Autodesk Fusion 360 part; units mm, degrees
note: some values were not read from the file. Chosen so that the rebuilt part matches the saved one: which face or edge a step refers to. Set by a fixed rule: which sketch regions a step uses.
(part 2 of 2)
sketch "Skizze1 (3)" plane through (0, 0, 8) normal (0, 0, 1) x (1, 0, 0) in component "Component''"
  arc A0 (-8, 3) -> (-3, -2) centre (-3, 3) ccw
  line L0 (-3, -2) -> (42, -2)
  arc A1 (42, -2) -> (47, 3) centre (42, 3) ccw
  line L1 (47, 3) -> (47, 46.6)
  arc A2 (47, 46.6) -> (42, 51.6) centre (42, 46.6) ccw
  line L2 (42, 51.6) -> (-3, 51.6)
  arc A3 (-3, 51.6) -> (-8, 46.6) centre (-3, 46.6) ccw
  line L3 (-8, 46.6) -> (-8, 3)
  circle A4 centre (42.5, 2.5) radius 1.5
  line L4 (36.6, 34.1) -> (36.1, 34.1)
  line L5 (36.1, 34.1) -> (36.1, 41.1)
  line L6 (36.1, 41.1) -> (28.8, 41.1)
  line L7 (28.8, 41.1) -> (28.8, 34.1)
  line L8 (28.8, 34.1) -> (28.3, 34.1)
  line L9 (28.3, 34.1) -> (28.3, 41.6)
  line L10 (28.3, 41.6) -> (36.6, 41.6)
  line L11 (36.6, 41.6) -> (36.6, 34.1)
  line L12 (27.1, 34.1) -> (26.6, 34.1)
  line L13 (26.6, 34.1) -> (26.6, 41.1)
  line L14 (26.6, 41.1) -> (19.3, 41.1)
  line L15 (19.3, 41.1) -> (19.3, 34.1)
  line L16 (19.3, 34.1) -> (18.8, 34.1)
  line L17 (18.8, 34.1) -> (18.8, 41.6)
  line L18 (18.8, 41.6) -> (27.1, 41.6)
  line L19 (27.1, 41.6) -> (27.1, 34.1)
  line L20 (17.6, 34.1) -> (17.1, 34.1)
  line L21 (17.1, 34.1) -> (17.1, 41.1)
  line L22 (17.1, 41.1) -> (9.8, 41.1)
  line L23 (9.8, 41.1) -> (9.8, 34.1)
  line L24 (9.8, 34.1) -> (9.3, 34.1)
  line L25 (9.3, 34.1) -> (9.3, 41.6)
  line L26 (9.3, 41.6) -> (17.6, 41.6)
  line L27 (17.6, 41.6) -> (17.6, 34.1)
  circle A5 centre (-3.5, 2.5) radius 1.5
  circle A6 centre (42.5, 47.1) radius 1.5
  circle A7 centre (-3.5, 47.1) radius 1.5
  line L28 (17.6, 7.6) -> (17.1, 7.6)
  line L29 (17.1, 7.6) -> (17.1, 14.6)
  line L30 (17.1, 14.6) -> (9.8, 14.6)
  line L31 (9.8, 14.6) -> (9.8, 7.6)
  line L32 (9.8, 7.6) -> (9.3, 7.6)
  line L33 (9.3, 7.6) -> (9.3, 15.1)
  line L34 (9.3, 15.1) -> (17.6, 15.1)
  line L35 (17.6, 15.1) -> (17.6, 7.6)
  line L36 (27.1, 7.6) -> (26.6, 7.6)
  line L37 (26.6, 7.6) -> (26.6, 14.6)
  line L38 (26.6, 14.6) -> (19.3, 14.6)
  line L39 (19.3, 14.6) -> (19.3, 7.6)
  line L40 (19.3, 7.6) -> (18.8, 7.6)
  line L41 (18.8, 7.6) -> (18.8, 15.1)
  line L42 (18.8, 15.1) -> (27.1, 15.1)
  line L43 (27.1, 15.1) -> (27.1, 7.6)
  line L44 (17.6, 25.2667) -> (17.1, 25.2667)
  line L45 (17.1, 25.2667) -> (17.1, 32.2667)
  line L46 (17.1, 32.2667) -> (9.8, 32.2667)
  line L47 (9.8, 32.2667) -> (9.8, 25.2667)
  line L48 (9.8, 25.2667) -> (9.3, 25.2667)
  line L49 (9.3, 25.2667) -> (9.3, 32.7667)
  line L50 (9.3, 32.7667) -> (17.6, 32.7667)
  line L51 (17.6, 32.7667) -> (17.6, 25.2667)
  line L52 (36.6, 7.6) -> (36.1, 7.6)
  line L53 (36.1, 7.6) -> (36.1, 14.6)
  line L54 (36.1, 14.6) -> (28.8, 14.6)
  line L55 (28.8, 14.6) -> (28.8, 7.6)
  line L56 (28.8, 7.6) -> (28.3, 7.6)
  line L57 (28.3, 7.6) -> (28.3, 15.1)
  line L58 (28.3, 15.1) -> (36.6, 15.1)
  line L59 (36.6, 15.1) -> (36.6, 7.6)
  line L60 (-0.2, 41.6) -> (8.1, 41.6)
  line L61 (8.1, 41.6) -> (8.1, 34.1)
  line L62 (8.1, 34.1) -> (7.6, 34.1)
  line L63 (7.6, 34.1) -> (7.6, 41.1)
  line L64 (7.6, 41.1) -> (0.3, 41.1)
  line L65 (0.3, 41.1) -> (0.3, 34.1)
  line L66 (0.3, 34.1) -> (-0.2, 34.1)
  line L67 (-0.2, 34.1) -> (-0.2, 41.6)
  line L68 (8.1, 25.2667) -> (7.6, 25.2667)
  line L69 (7.6, 25.2667) -> (7.6, 32.2667)
  line L70 (7.6, 32.2667) -> (0.3, 32.2667)
  line L71 (0.3, 32.2667) -> (0.3, 25.2667)
  line L72 (0.3, 25.2667) -> (-0.2, 25.2667)
  line L73 (-0.2, 25.2667) -> (-0.2, 32.7667)
  line L74 (-0.2, 32.7667) -> (8.1, 32.7667)
  line L75 (8.1, 32.7667) -> (8.1, 25.2667)
  line L76 (8.1, 16.4333) -> (7.6, 16.4333)
  line L77 (7.6, 16.4333) -> (7.6, 23.4333)
  line L78 (7.6, 23.4333) -> (0.3, 23.4333)
  line L79 (0.3, 23.4333) -> (0.3, 16.4333)
  line L80 (0.3, 16.4333) -> (-0.2, 16.4333)
  line L81 (-0.2, 16.4333) -> (-0.2, 23.9333)
  line L82 (-0.2, 23.9333) -> (8.1, 23.9333)
  line L83 (8.1, 23.9333) -> (8.1, 16.4333)
  line L84 (8.1, 7.6) -> (7.6, 7.6)
  line L85 (7.6, 7.6) -> (7.6, 14.6)
  line L86 (7.6, 14.6) -> (0.3, 14.6)
  line L87 (0.3, 14.6) -> (0.3, 7.6)
  line L88 (0.3, 7.6) -> (-0.2, 7.6)
  line L89 (-0.2, 7.6) -> (-0.2, 15.1)
  line L90 (-0.2, 15.1) -> (8.1, 15.1)
  line L91 (8.1, 15.1) -> (8.1, 7.6)
  line L92 (36.6, 16.4333) -> (36.1, 16.4333)
  line L93 (36.1, 16.4333) -> (36.1, 23.4333)
  line L94 (36.1, 23.4333) -> (28.8, 23.4333)
  line L95 (28.8, 23.4333) -> (28.8, 16.4333)
  line L96 (28.8, 16.4333) -> (28.3, 16.4333)
  line L97 (28.3, 16.4333) -> (28.3, 23.9333)
  line L98 (28.3, 23.9333) -> (36.6, 23.9333)
  line L99 (36.6, 23.9333) -> (36.6, 16.4333)
  line L100 (27.1, 16.4333) -> (26.6, 16.4333)
  line L101 (26.6, 16.4333) -> (26.6, 23.4333)
  line L102 (26.6, 23.4333) -> (19.3, 23.4333)
  line L103 (19.3, 23.4333) -> (19.3, 16.4333)
  line L104 (19.3, 16.4333) -> (18.8, 16.4333)
  line L105 (18.8, 16.4333) -> (18.8, 23.9333)
  line L106 (18.8, 23.9333) -> (27.1, 23.9333)
  line L107 (27.1, 23.9333) -> (27.1, 16.4333)
  line L108 (17.6, 16.4333) -> (17.1, 16.4333)
  line L109 (17.1, 16.4333) -> (17.1, 23.4333)
  line L110 (17.1, 23.4333) -> (9.8, 23.4333)
  line L111 (9.8, 23.4333) -> (9.8, 16.4333)
  line L112 (9.8, 16.4333) -> (9.3, 16.4333)
  line L113 (9.3, 16.4333) -> (9.3, 23.9333)
  line L114 (9.3, 23.9333) -> (17.6, 23.9333)
  line L115 (17.6, 23.9333) -> (17.6, 16.4333)
  line L116 (36.6, 25.2667) -> (36.1, 25.2667)
  line L117 (36.1, 25.2667) -> (36.1, 32.2667)
  line L118 (36.1, 32.2667) -> (28.8, 32.2667)
  line L119 (28.8, 32.2667) -> (28.8, 25.2667)
  line L120 (28.8, 25.2667) -> (28.3, 25.2667)
  line L121 (28.3, 25.2667) -> (28.3, 32.7667)
  line L122 (28.3, 32.7667) -> (36.6, 32.7667)
  line L123 (36.6, 32.7667) -> (36.6, 25.2667)
  line L124 (27.1, 25.2667) -> (26.6, 25.2667)
  line L125 (26.6, 25.2667) -> (26.6, 32.2667)
  line L126 (26.6, 32.2667) -> (19.3, 32.2667)
  line L127 (19.3, 32.2667) -> (19.3, 25.2667)
  line L128 (19.3, 25.2667) -> (18.8, 25.2667)
  line L129 (18.8, 25.2667) -> (18.8, 32.7667)
  line L130 (18.8, 32.7667) -> (27.1, 32.7667)
  line L131 (27.1, 32.7667) -> (27.1, 25.2667)
extrude "Extrusion1''" add sketch "Skizze1 (3)" along normal blind 1.5 separate body makes body 5 in component "Component''"
sketch "Skizze2 (3)" plane through (0, 0, 9.5) normal (0, 0, 1) x (1, 0, 0) in component "Component''"
  line L0 (28.3, 15.1) -> (36.6, 15.1)
  line L1 (36.6, 15.1) -> (36.6, 7.6)
  line L2 (36.6, 7.6) -> (36.1, 7.6)
  line L3 (36.1, 7.6) -> (36.1, 14.6)
  line L4 (36.1, 14.6) -> (28.8, 14.6)
  line L5 (28.8, 14.6) -> (28.8, 7.6)
  line L6 (28.8, 7.6) -> (28.3, 7.6)
  line L7 (28.3, 7.6) -> (28.3, 15.1)
  line L8 (28.3, 32.7667) -> (36.6, 32.7667)
  line L9 (36.6, 32.7667) -> (36.6, 25.2667)
  line L10 (36.6, 25.2667) -> (36.1, 25.2667)
  line L11 (36.1, 25.2667) -> (36.1, 32.2667)
  line L12 (36.1, 32.2667) -> (28.8, 32.2667)
  line L13 (28.8, 32.2667) -> (28.8, 25.2667)
  line L14 (28.8, 25.2667) -> (28.3, 25.2667)
  line L15 (28.3, 25.2667) -> (28.3, 32.7667)
  line L16 (28.3, 23.9333) -> (36.6, 23.9333)
  line L17 (36.6, 23.9333) -> (36.6, 16.4333)
  line L18 (36.6, 16.4333) -> (36.1, 16.4333)
  line L19 (36.1, 16.4333) -> (36.1, 23.4333)
  line L20 (36.1, 23.4333) -> (28.8, 23.4333)
  line L21 (28.8, 23.4333) -> (28.8, 16.4333)
  line L22 (28.8, 16.4333) -> (28.3, 16.4333)
  line L23 (28.3, 16.4333) -> (28.3, 23.9333)
  line L24 (9.3, 32.7667) -> (17.6, 32.7667)
  line L25 (17.6, 32.7667) -> (17.6, 25.2667)
  line L26 (17.6, 25.2667) -> (17.1, 25.2667)
  line L27 (17.1, 25.2667) -> (17.1, 32.2667)
  line L28 (17.1, 32.2667) -> (9.8, 32.2667)
  line L29 (9.8, 32.2667) -> (9.8, 25.2667)
  line L30 (9.8, 25.2667) -> (9.3, 25.2667)
  line L31 (9.3, 25.2667) -> (9.3, 32.7667)
  line L32 (18.8, 15.1) -> (27.1, 15.1)
  line L33 (27.1, 15.1) -> (27.1, 7.6)
  line L34 (27.1, 7.6) -> (26.6, 7.6)
  line L35 (26.6, 7.6) -> (26.6, 14.6)
  line L36 (26.6, 14.6) -> (19.3, 14.6)
  line L37 (19.3, 14.6) -> (19.3, 7.6)
  line L38 (19.3, 7.6) -> (18.8, 7.6)
  line L39 (18.8, 7.6) -> (18.8, 15.1)
  line L40 (18.8, 32.7667) -> (27.1, 32.7667)
  line L41 (27.1, 32.7667) -> (27.1, 25.2667)
  line L42 (27.1, 25.2667) -> (26.6, 25.2667)
  line L43 (26.6, 25.2667) -> (26.6, 32.2667)
  line L44 (26.6, 32.2667) -> (19.3, 32.2667)
  line L45 (19.3, 32.2667) -> (19.3, 25.2667)
  line L46 (19.3, 25.2667) -> (18.8, 25.2667)
  line L47 (18.8, 25.2667) -> (18.8, 32.7667)
  circle A0 centre (-3.5, 2.5) radius 1.5
  line L48 (9.3, 15.1) -> (17.6, 15.1)
  line L49 (17.6, 15.1) -> (17.6, 7.6)
  line L50 (17.6, 7.6) -> (17.1, 7.6)
  line L51 (17.1, 7.6) -> (17.1, 14.6)
  line L52 (17.1, 14.6) -> (9.8, 14.6)
  line L53 (9.8, 14.6) -> (9.8, 7.6)
  line L54 (9.8, 7.6) -> (9.3, 7.6)
  line L55 (9.3, 7.6) -> (9.3, 15.1)
  line L56 (-0.2, 32.7667) -> (8.1, 32.7667)
  line L57 (8.1, 32.7667) -> (8.1, 25.2667)
  line L58 (8.1, 25.2667) -> (7.6, 25.2667)
  line L59 (7.6, 25.2667) -> (7.6, 32.2667)
  line L60 (7.6, 32.2667) -> (0.3, 32.2667)
  line L61 (0.3, 32.2667) -> (0.3, 25.2667)
  line L62 (0.3, 25.2667) -> (-0.2, 25.2667)
  line L63 (-0.2, 25.2667) -> (-0.2, 32.7667)
  line L64 (-0.2, 15.1) -> (8.1, 15.1)
  line L65 (8.1, 15.1) -> (8.1, 7.6)
  line L66 (8.1, 7.6) -> (7.6, 7.6)
  line L67 (7.6, 7.6) -> (7.6, 14.6)
  line L68 (7.6, 14.6) -> (0.3, 14.6)
  line L69 (0.3, 14.6) -> (0.3, 7.6)
  line L70 (0.3, 7.6) -> (-0.2, 7.6)
  line L71 (-0.2, 7.6) -> (-0.2, 15.1)
  line L72 (18.8, 23.9333) -> (27.1, 23.9333)
  line L73 (27.1, 23.9333) -> (27.1, 16.4333)
  line L74 (27.1, 16.4333) -> (26.6, 16.4333)
  line L75 (26.6, 16.4333) -> (26.6, 23.4333)
  line L76 (26.6, 23.4333) -> (19.3, 23.4333)
  line L77 (19.3, 23.4333) -> (19.3, 16.4333)
  line L78 (19.3, 16.4333) -> (18.8, 16.4333)
  line L79 (18.8, 16.4333) -> (18.8, 23.9333)
  line L80 (28.3, 41.6) -> (36.6, 41.6)
  line L81 (36.6, 41.6) -> (36.6, 34.1)
  line L82 (36.6, 34.1) -> (36.1, 34.1)
  line L83 (36.1, 34.1) -> (36.1, 41.1)
  line L84 (36.1, 41.1) -> (28.8, 41.1)
  line L85 (28.8, 41.1) -> (28.8, 34.1)
  line L86 (28.8, 34.1) -> (28.3, 34.1)
  line L87 (28.3, 34.1) -> (28.3, 41.6)
  line L88 (9.3, 41.6) -> (17.6, 41.6)
  line L89 (17.6, 41.6) -> (17.6, 34.1)
  line L90 (17.6, 34.1) -> (17.1, 34.1)
  line L91 (17.1, 34.1) -> (17.1, 41.1)
  line L92 (17.1, 41.1) -> (9.8, 41.1)
  line L93 (9.8, 41.1) -> (9.8, 34.1)
  line L94 (9.8, 34.1) -> (9.3, 34.1)
  line L95 (9.3, 34.1) -> (9.3, 41.6)
  line L96 (18.8, 41.6) -> (27.1, 41.6)
  line L97 (27.1, 41.6) -> (27.1, 34.1)
  line L98 (27.1, 34.1) -> (26.6, 34.1)
  line L99 (26.6, 34.1) -> (26.6, 41.1)
  line L100 (26.6, 41.1) -> (19.3, 41.1)
  line L101 (19.3, 41.1) -> (19.3, 34.1)
  line L102 (19.3, 34.1) -> (18.8, 34.1)
  line L103 (18.8, 34.1) -> (18.8, 41.6)
  circle A1 centre (42.5, 47.1) radius 1.5
  line L104 (-0.2, 23.9333) -> (8.1, 23.9333)
  line L105 (8.1, 23.9333) -> (8.1, 16.4333)
  line L106 (8.1, 16.4333) -> (7.6, 16.4333)
  line L107 (7.6, 16.4333) -> (7.6, 23.4333)
  line L108 (7.6, 23.4333) -> (0.3, 23.4333)
  line L109 (0.3, 23.4333) -> (0.3, 16.4333)
  line L110 (0.3, 16.4333) -> (-0.2, 16.4333)
  line L111 (-0.2, 16.4333) -> (-0.2, 23.9333)
  circle A2 centre (-3.5, 47.1) radius 1.5
  line L112 (0.3, 34.1) -> (-0.2, 34.1)
  line L113 (-0.2, 34.1) -> (-0.2, 41.6)
  line L114 (-0.2, 41.6) -> (8.1, 41.6)
  line L115 (8.1, 41.6) -> (8.1, 34.1)
  line L116 (8.1, 34.1) -> (7.6, 34.1)
  line L117 (7.6, 34.1) -> (7.6, 41.1)
  line L118 (7.6, 41.1) -> (0.3, 41.1)
  line L119 (0.3, 41.1) -> (0.3, 34.1)
  circle A3 centre (42.5, 2.5) radius 1.5
  line L120 (9.3, 23.9333) -> (17.6, 23.9333)
  line L121 (17.6, 23.9333) -> (17.6, 16.4333)
  line L122 (17.6, 16.4333) -> (17.1, 16.4333)
  line L123 (17.1, 16.4333) -> (17.1, 23.4333)
  line L124 (17.1, 23.4333) -> (9.8, 23.4333)
  line L125 (9.8, 23.4333) -> (9.8, 16.4333)
  line L126 (9.8, 16.4333) -> (9.3, 16.4333)
  line L127 (9.3, 16.4333) -> (9.3, 23.9333)
  line L128 (-8, 46.6) -> (-8, 3)
  arc A4 (-8, 3) -> (-3, -2) centre (-3, 3) ccw
  line L129 (-3, -2) -> (42, -2)
  arc A5 (42, -2) -> (47, 3) centre (42, 3) ccw
  line L130 (47, 3) -> (47, 46.6)
  arc A6 (47, 46.6) -> (42, 51.6) centre (42, 46.6) ccw
  line L131 (42, 51.6) -> (-3, 51.6)
  arc A7 (-3, 51.6) -> (-8, 46.6) centre (-3, 46.6) ccw
  line L132 (0.3, 41.1) -> (7.6, 41.1)
  line L133 (7.6, 41.1) -> (7.6, 34.1)
  line L134 (7.6, 34.1) -> (0.3, 34.1)
  line L135 (0.3, 34.1) -> (0.3, 41.1)
  line L136 (9.8, 41.1) -> (9.8, 34.1)
  line L137 (17.1, 41.1) -> (17.1, 34.1)
  line L138 (17.1, 34.1) -> (9.8, 34.1)
  line L139 (9.8, 41.1) -> (17.1, 41.1)
  line L140 (17.1, 34.1) -> (17.1, 41.1)
  line L141 (9.8, 34.1) -> (9.8, 41.1)
  line L142 (17.1, 41.1) -> (9.8, 41.1)
  line L143 (19.3, 41.1) -> (19.3, 34.1)
  line L144 (26.6, 41.1) -> (26.6, 34.1)
  line L145 (26.6, 34.1) -> (19.3, 34.1)
  line L146 (19.3, 41.1) -> (26.6, 41.1)
  line L147 (26.6, 34.1) -> (26.6, 41.1)
  line L148 (19.3, 34.1) -> (19.3, 41.1)
  line L149 (26.6, 41.1) -> (19.3, 41.1)
  line L150 (28.8, 41.1) -> (28.8, 34.1)
  line L151 (36.1, 41.1) -> (36.1, 34.1)
  line L152 (36.1, 34.1) -> (28.8, 34.1)
  line L153 (28.8, 41.1) -> (36.1, 41.1)
  line L154 (36.1, 34.1) -> (36.1, 41.1)
  line L155 (28.8, 34.1) -> (28.8, 41.1)
  line L156 (36.1, 41.1) -> (28.8, 41.1)
  line L157 (0.3, 32.2667) -> (0.3, 25.2667)
  line L158 (7.6, 32.2667) -> (7.6, 25.2667)
  line L159 (7.6, 25.2667) -> (0.3, 25.2667)
  line L160 (0.3, 32.2667) -> (7.6, 32.2667)
  line L161 (7.6, 25.2667) -> (7.6, 32.2667)
  line L162 (0.3, 25.2667) -> (0.3, 32.2667)
  line L163 (7.6, 32.2667) -> (0.3, 32.2667)
  line L164 (9.8, 32.2667) -> (9.8, 25.2667)
  line L165 (17.1, 32.2667) -> (17.1, 25.2667)
  line L166 (17.1, 25.2667) -> (9.8, 25.2667)
  line L167 (9.8, 32.2667) -> (17.1, 32.2667)
  line L168 (17.1, 25.2667) -> (17.1, 32.2667)
  line L169 (9.8, 25.2667) -> (9.8, 32.2667)
  line L170 (17.1, 32.2667) -> (9.8, 32.2667)
  line L171 (19.3, 32.2667) -> (19.3, 25.2667)
  line L172 (26.6, 32.2667) -> (26.6, 25.2667)
  line L173 (26.6, 25.2667) -> (19.3, 25.2667)
  line L174 (19.3, 32.2667) -> (26.6, 32.2667)
  line L175 (26.6, 25.2667) -> (26.6, 32.2667)
  line L176 (19.3, 25.2667) -> (19.3, 32.2667)
  line L177 (26.6, 32.2667) -> (19.3, 32.2667)
  line L178 (28.8, 32.2667) -> (28.8, 25.2667)
  line L179 (36.1, 32.2667) -> (36.1, 25.2667)
  line L180 (36.1, 25.2667) -> (28.8, 25.2667)
  line L181 (28.8, 32.2667) -> (36.1, 32.2667)
  line L182 (36.1, 25.2667) -> (36.1, 32.2667)
  line L183 (28.8, 25.2667) -> (28.8, 32.2667)
  line L184 (36.1, 32.2667) -> (28.8, 32.2667)
  line L185 (0.3, 23.4333) -> (0.3, 16.4333)
  line L186 (7.6, 23.4333) -> (7.6, 16.4333)
  line L187 (7.6, 16.4333) -> (0.3, 16.4333)
  line L188 (0.3, 23.4333) -> (7.6, 23.4333)
  line L189 (7.6, 16.4333) -> (7.6, 23.4333)
  line L190 (0.3, 16.4333) -> (0.3, 23.4333)
  line L191 (7.6, 23.4333) -> (0.3, 23.4333)
  line L192 (9.8, 23.4333) -> (9.8, 16.4333)
  line L193 (17.1, 23.4333) -> (17.1, 16.4333)
  line L194 (17.1, 16.4333) -> (9.8, 16.4333)
  line L195 (9.8, 23.4333) -> (17.1, 23.4333)
  line L196 (17.1, 16.4333) -> (17.1, 23.4333)
  line L197 (9.8, 16.4333) -> (9.8, 23.4333)
  line L198 (17.1, 23.4333) -> (9.8, 23.4333)
  line L199 (19.3, 23.4333) -> (19.3, 16.4333)
  line L200 (26.6, 23.4333) -> (26.6, 16.4333)
  line L201 (26.6, 16.4333) -> (19.3, 16.4333)
  line L202 (19.3, 23.4333) -> (26.6, 23.4333)
  line L203 (26.6, 16.4333) -> (26.6, 23.4333)
  line L204 (19.3, 16.4333) -> (19.3, 23.4333)
  line L205 (26.6, 23.4333) -> (19.3, 23.4333)
  line L206 (28.8, 23.4333) -> (28.8, 16.4333)
  line L207 (36.1, 23.4333) -> (36.1, 16.4333)
  line L208 (36.1, 16.4333) -> (28.8, 16.4333)
  line L209 (28.8, 23.4333) -> (36.1, 23.4333)
  line L210 (36.1, 16.4333) -> (36.1, 23.4333)
  line L211 (28.8, 16.4333) -> (28.8, 23.4333)
  line L212 (36.1, 23.4333) -> (28.8, 23.4333)
  line L213 (0.3, 14.6) -> (0.3, 7.6)
  line L214 (7.6, 14.6) -> (7.6, 7.6)
  line L215 (7.6, 7.6) -> (0.3, 7.6)
  line L216 (0.3, 14.6) -> (7.6, 14.6)
  line L217 (7.6, 7.6) -> (7.6, 14.6)
  line L218 (0.3, 7.6) -> (0.3, 14.6)
  line L219 (7.6, 14.6) -> (0.3, 14.6)
  line L220 (9.8, 14.6) -> (9.8, 7.6)
  line L221 (17.1, 14.6) -> (17.1, 7.6)
  line L222 (17.1, 7.6) -> (9.8, 7.6)
  line L223 (9.8, 14.6) -> (17.1, 14.6)
  line L224 (17.1, 7.6) -> (17.1, 14.6)
  line L225 (9.8, 7.6) -> (9.8, 14.6)
  line L226 (17.1, 14.6) -> (9.8, 14.6)
  line L227 (19.3, 14.6) -> (19.3, 7.6)
  line L228 (26.6, 14.6) -> (26.6, 7.6)
  line L229 (26.6, 7.6) -> (19.3, 7.6)
  line L230 (19.3, 14.6) -> (26.6, 14.6)
  line L231 (26.6, 7.6) -> (26.6, 14.6)
  line L232 (19.3, 7.6) -> (19.3, 14.6)
  line L233 (26.6, 14.6) -> (19.3, 14.6)
  line L234 (28.8, 14.6) -> (28.8, 7.6)
  line L235 (36.1, 14.6) -> (36.1, 7.6)
  line L236 (36.1, 7.6) -> (28.8, 7.6)
  line L237 (28.8, 14.6) -> (36.1, 14.6)
  line L238 (36.1, 7.6) -> (36.1, 14.6)
  line L239 (28.8, 7.6) -> (28.8, 14.6)
  line L240 (36.1, 14.6) -> (28.8, 14.6)
  dimension "d347" = 28.5
  dimension "d348" = -26.5
extrude "Extrusion2'" add sketch "Skizze2 (3)" along normal blind 3 contours L3 L4 L5 L234 L235 L236 L237 L238 L239 L240 | L11 L12 L13 L178 L179 L180 L181 L182 L183 L184 | L19 L20 L21 L206 L207 L208 L209 L210 L211 L212 | L27 L28 L29 L164 L165 L166 L167 L168 L169 L170 | L35 L36 L37 L227 L228 L229 L230 L231 L232 L233 | L43 L44 L45 L171 L172 L173 L174 L175 L176 L177 | L51 L52 L53 L220 L221 L222 L223 L224 L225 L226 | L59 L60 L61 L157 L158 L159 L160 L161 L162 L163 | L67 L68 L69 L213 L214 L215 L216 L217 L218 L219 | L75 L76 L77 L199 L200 L201 L202 L203 L204 L205 | L83 L84 L85 L150 L151 L152 L153 L154 L155 L156 | L91 L92 L93 L136 L137 L138 L139 L140 L141 L142 | L99 L100 L101 L143 L144 L145 L146 L147 L148 L149 | L107 L108 L109 L185 L186 L187 L188 L189 L190 L191 | L117 L118 L119 L132 L133 L134 L135 | L123 L124 L125 L192 L193 L194 L195 L196 L197 L198 bodies 5 in component "Component''"
chamfer "Fase1" distance 1.5 angle 45 64 edges at (0.3, 37.6, 12.5) (3.95, 41.1, 12.5) (7.6, 37.6, 12.5) (3.95, 34.1, 12.5) (9.8, 37.6, 12.5) (13.45, 41.1, 12.5) (17.1, 37.6, 12.5) (13.45, 34.1, 12.5) (19.3, 37.6, 12.5) (22.95, 41.1, 12.5) (26.6, 37.6, 12.5) (22.95, 34.1, 12.5) (28.8, 37.6, 12.5) (32.45, 41.1, 12.5) (36.1, 37.6, 12.5) (32.45, 34.1, 12.5) (0.3, 28.7667, 12.5) (3.95, 32.2667, 12.5) (7.6, 28.7667, 12.5) (3.95, 25.2667, 12.5) (9.8, 28.7667, 12.5) (13.45, 32.2667, 12.5) (17.1, 28.7667, 12.5) (13.45, 25.2667, 12.5) (19.3, 28.7667, 12.5) (22.95, 32.2667, 12.5) (26.6, 28.7667, 12.5) (22.95, 25.2667, 12.5) (28.8, 28.7667, 12.5) (32.45, 32.2667, 12.5) (36.1, 28.7667, 12.5) (32.45, 25.2667, 12.5) (0.3, 19.9333, 12.5) (3.95, 23.4333, 12.5) (7.6, 19.9333, 12.5) (3.95, 16.4333, 12.5) (9.8, 19.9333, 12.5) (13.45, 23.4333, 12.5) (17.1, 19.9333, 12.5) (13.45, 16.4333, 12.5) (19.3, 19.9333, 12.5) (22.95, 23.4333, 12.5) (26.6, 19.9333, 12.5) (22.95, 16.4333, 12.5) (28.8, 19.9333, 12.5) (32.45, 23.4333, 12.5) (36.1, 19.9333, 12.5) (32.45, 16.4333, 12.5) (0.3, 11.1, 12.5) (3.95, 14.6, 12.5) (7.6, 11.1, 12.5) (3.95, 7.6, 12.5) (9.8, 11.1, 12.5) (13.45, 14.6, 12.5) (17.1, 11.1, 12.5) (13.45, 7.6, 12.5) (19.3, 11.1, 12.5) (22.95, 14.6, 12.5) (26.6, 11.1, 12.5) (22.95, 7.6, 12.5) (28.8, 11.1, 12.5) (32.45, 14.6, 12.5) (36.1, 11.1, 12.5) (32.45, 7.6, 12.5) on bodies 5 in component "Component''"
component "Component" placed x (1, 0, 0) y (0, 1, 0) z (0, 0, 1) at (0, 0, 0)
component "Component'" placed x (1, 0, 0) y (0, 1, 0) z (0, 0, 1) at (0, 0, 0)
component "Component''" placed x (1, 0, 0) y (0, 1, 0) z (0, 0, 1) at (0, 0, 0)
equation "d277 = ( 5.6 / 2 ) * 1 mm"
